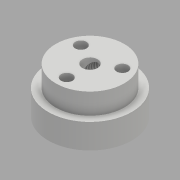
# Autodesk Inventor part: WheelAdapter-4mm
Saved by Autodesk Inventor 2017 (Build 210142000, 142)
## iProperties
Created: 2017-05-07
Part Number: WheelAdapter-4mm
Material: Generic
Document SubType Name: Modeling
Designer: zallen
Density: 1 g/cm^3
Appearance: Default
Author: zallen
Autodesk Inventor part; units mm, degrees
ref_plane "YZ Plane" through (0, 0, 0) normal (1, 0, 0) x (0, 1, 0)
ref_plane "XZ Plane" through (0, 0, 0) normal (0, 1, 0) x (-1, 0, 0)
ref_plane "XY Plane" through (0, 0, 0) normal (0, 0, 1) x (1, 0, 0)
sketch "Sketch1" plane through (0, 0, 0) normal (0, 0, 1) x (1, 0, 0)
  circle A0 centre (0, 0) radius 11
  circle A1 centre (0, 0) radius 2
  dimension "d0" = 22
  dimension "d1" = 4
  constraints: 2 centre point, 2 coincident
  measures "d0" diameter of A0
  measures "d1" diameter of A1
extrude "Extrusion1" add sketch "Sketch1" along normal blind 6.5
sketch "Sketch2" plane through (0, 0, 6.5) normal (0, 0, 1) x (1, 0, 0)
  circle A0 centre (0, 0) radius 9
  circle A1 centre (0, 0) radius 2
  dimension "d4" = 18
  constraints: 2 centre point, 2 coincident
  measures "d4" diameter of A0
extrude "Extrusion2" add sketch "Sketch2" along normal blind 5.5
sketch "Sketch3" plane through (0, 0, 12) normal (0, 0, 1) x (1, 0, 0)
  circle A0 centre (-5.4177, 3.0147) radius 1.5
  circle A1 centre (0.098, -6.1992) radius 1.5
  circle A2 centre (5.3197, 3.1845) radius 1.5
  circle A3 centre (0, 0) radius 6.2 construction
  dimension "d21" = 12.4
  dimension "d7" = 3
  dimension "d10" = 360
  constraints: 3 centre point, 1 coincident, 10 other
  measures "d7" diameter of A0
extrude "Extrusion3" cut sketch "Sketch3" against normal through all
sketch "Sketch4" plane through (0, 0, 0) normal (0, 1, 0) x (-1, 0, 0)
  circle A0 centre (0, 9.25) radius 2
  circle A1 centre (0, 3.25) radius 2
  line L0 (0, 0) -> (0, 21.1328) construction
  dimension "d15" = 4
  dimension "d16" = 4
  dimension "d17" = 3.25
  dimension "d18" = 9.25
  constraints: 2 centre point, 2 end point, 2 point on line, 1 vertical
  measures "d15" diameter of A0
  measures "d16" diameter of A1
  measures "d17" distance of L0.start A1.centre
  measures "d18" distance of L0.start A0.centre
extrude "Extrusion4" cut sketch "Sketch4" along normal through all
thread "Thread1" size "M4x0.7" class "6H" standard "ISO Metric profile" full length
thread "Thread2" size "M4x0.7" class "6H" standard "ISO Metric profile" full length
body "Solid1"
